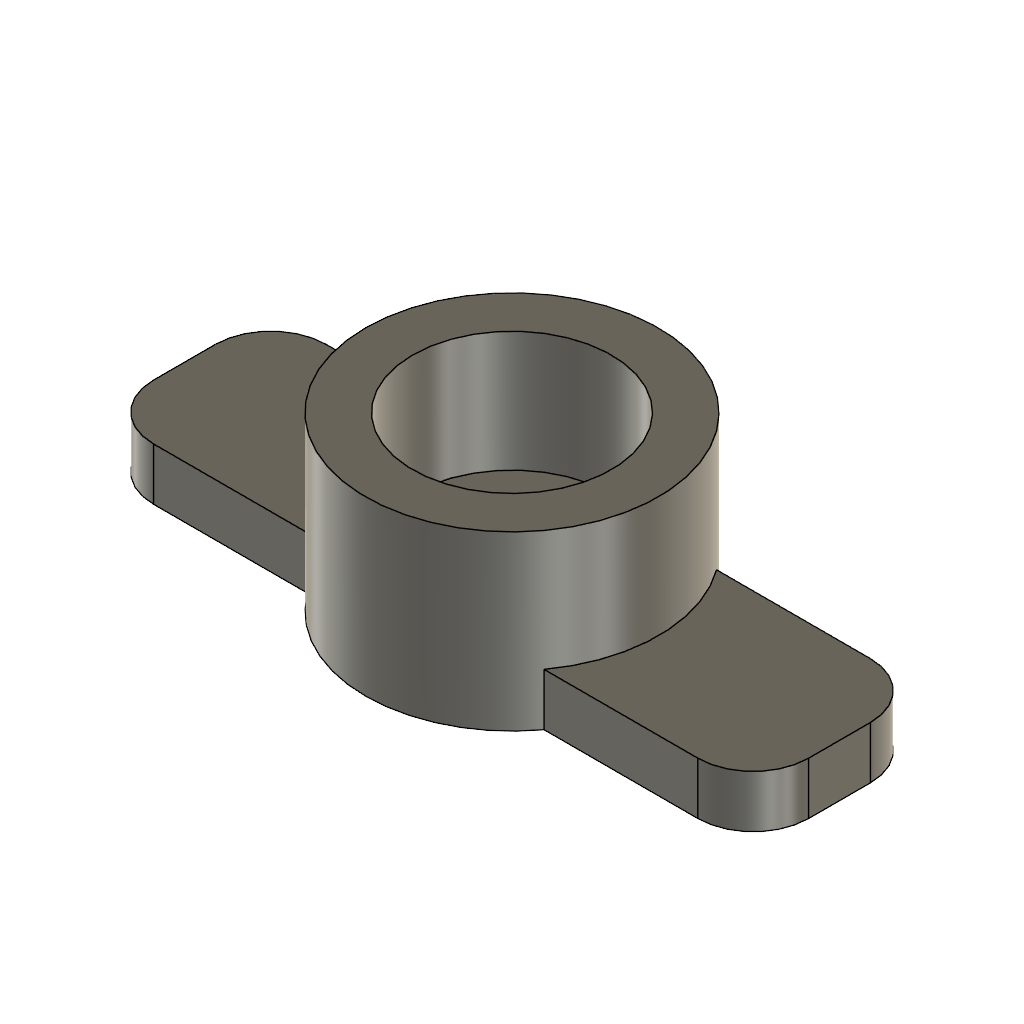
gear pan s0.95 (Autodesk Fusion 360 archive; units mm, degrees)
design "horn"
Autodesk Fusion 360 part; units mm, degrees
sketch "Boceto1" plane through (0, 0, 0) normal (0, 0, 1) x (1, 0, 0)
  circle A0 centre (0, 0) radius 2.8
  line L0 (-6.2622, 1.65) -> (6.2622, 1.65)
  line L1 (6.2622, 1.65) -> (6.2622, -1.65)
  line L2 (6.2622, -1.65) -> (-6.2622, -1.65)
  line L3 (-6.2622, -1.65) -> (-6.2622, 1.65)
  line L4 (-6.2622, 0) -> (6.2622, 0) construction
  line L5 (0, 1.65) -> (0, 0) construction
  circle A1 centre (0, 0) radius 0.75
  circle A2 centre (0, 0) radius 1.9
  point P0 (2.2622, 1.65)
  dimension "d1" = 5.6
  dimension "d2" = 3.3
  dimension "d3" = 4
  dimension "d8" = 1.5
  dimension "d9" = 3.8
  constraint coincident A0.centre L5.end
  constraint horizontal L0
  constraint vertical L1
  constraint horizontal L2
  constraint vertical L3
  constraint midpoint L3 L4.start
  constraint midpoint L1 L4.end
  constraint midpoint L0 L5.start
  constraint midpoint L4 A0.centre
  constraint coincident A0 P0
  constraint coincident L0 P0
  measures "d1" diameter of A0
  measures "d2" distance of L0 L2
  measures "d3" distance of L1 P0
  measures "d8" diameter of A1
  measures "d9" diameter of A2
extrude "Extruir1" add sketch "Boceto1" along normal blind 1 contours A0 L0 L2 A2 | A0 L0 L1 L2 | A0 L0 L2 A2 | A0 L0 L2 L3 | L0 L2 A2
extrude "Extruir2" add sketch "Boceto1" along normal blind 3.3 contours A0 L0 L2 A2 | A0 L0 A2 | A0 L2 A2 | A0 L0 L2 A2 | L0 L2 A2 | L0 A2 | L2 A2
extrude "Extruir3" cut sketch "Boceto1" along normal through all from surface at 1 contours L0 L2 A2 | L0 A2 | L2 A2
fillet "Empalme1" radius 1.059 4 edges at (-6.2622, 1.65, 0.5) (-6.2622, -1.65, 0.5) (6.2622, 1.65, 0.5) (6.2622, -1.65, 0.5)
